Laptop Lift (Autodesk Fusion 360 design; units mm, degrees)
Autodesk Fusion 360 part; units mm, degrees
sketch "Sketch1" plane through (0, 0, 0) normal (0, 0, 1) x (1, 0, 0)
  line L0 (0, 0) -> (215, 0)
  line L1 (215, 0) -> (215, 180)
  line L2 (215, 180) -> (0, 180)
  line L3 (0, 180) -> (0, 0)
  line L4 (-17.5, 180) -> (232.5, 180)
  line L5 (232.5, 180) -> (232.5, 0)
  line L6 (232.5, 0) -> (-17.5, 0)
  line L7 (-17.5, 0) -> (-17.5, 180)
  line L8 (-17.5, 0) -> (0, 180)
  line L9 (232.5, 0) -> (215, 180)
  dimension "d1" = 215
  dimension "d2" = 180
  dimension "d3" = 250
  dimension "d4" = 180
  constraint horizontal L0
  constraint vertical L1
  constraint horizontal L2
  constraint vertical L3
  constraint coincident L0.start L3.end
  constraint horizontal L4
  constraint vertical L5
  constraint horizontal L6
  constraint vertical L7
  constraint collinear L2 L4
  constraint midpoint L0 L6
  measures "d1" distance of L1.end L2.end
  measures "d2" distance of L0.start L2.end
  measures "d3" distance of L4.start L4.end
  measures "d4" distance of L4.start L6.end
extrude "Extrude1" add sketch "Sketch1" along normal blind 3 contours L0 L1 L2 L3 L4 L6 | L3 L6 L8 | L1 L6 L9 makes body 1
fillet "Fillet1" radius 25 2 edges at (232.5, 0, 1.5) (-17.5, 0, 1.5) on bodies 1
sketch "Sketch5" plane through (0, 0, 3) normal (0, 0, 1) x (-1, 0, 0)
  arc A0 (14.8342, -27.4191) -> (-10.0484, 0) centre (-10.0484, -25) ccw
  line L0 (-10.0484, 0) -> (-204.9516, 0)
  arc A1 (-204.9516, 0) -> (-229.8342, -27.4191) centre (-204.9516, -25) ccw
  line L1 (-229.8342, -27.4191) -> (-215, -180)
  line L2 (-215, -180) -> (0, -180)
  line L3 (0, -180) -> (14.8342, -27.4191)
  arc A2 (17.8202, -27.7094) -> (-10.0484, 3) centre (-10.0484, -25) ccw
  line L4 (-10.0484, 3) -> (-204.9516, 3)
  arc A3 (-204.9516, 3) -> (-232.8202, -27.7094) centre (-204.9516, -25) ccw
  line L5 (-232.8202, -27.7094) -> (-217.7225, -183)
  line L6 (-217.7225, -183) -> (2.7225, -183)
  line L7 (2.7225, -183) -> (17.8202, -27.7094)
  line L8 (40, -180) -> (-310, -180)
  dimension "d21" = 3
  constraint horizontal L8
  constraint collinear L2 L8
extrude "Extrude4" add sketch "Sketch5" along normal blind 5 and the other way blind 3 contours A0 L0 A1 L1 L3 A2 L4 A3 L5 L7 L8 bodies 1
chamfer "Chamfer2" distance 80 distance2 4 2 edges at (216.5071, 180, 8) (-1.5071, 180, 8) measured on face at (75.0161, -1, 8) measured on face at (75.0161, -1, 8) on bodies 1
sketch "Sketch7" plane through (0, 0, 0) normal (0, 0, -1) x (1, 0, 0)
  line L0 (-3.0141, -180) -> (218.0141, -180)
  line L1 (218.0141, -180) -> (232.8202, -27.7094)
  arc A0 (232.8202, -27.7094) -> (204.9516, 3) centre (204.9516, -25) ccw
  line L2 (204.9516, 3) -> (10.0484, 3)
  arc A1 (10.0484, 3) -> (-17.8202, -27.7094) centre (10.0484, -25) ccw
  line L3 (-17.8202, -27.7094) -> (-3.0141, -180)
  line L4 (22, 3) -> (62, 3)
  line L5 (62, 3) -> (62, -147)
  line L6 (62, -147) -> (22, -147)
  line L7 (22, -147) -> (22, 3)
  line L8 (34.5, -122) -> (49.5, -122)
  line L9 (49.5, -122) -> (49.5, -107)
  line L10 (49.5, -107) -> (34.5, -107)
  line L11 (34.5, -107) -> (34.5, -122)
  line L12 (34.5, -82) -> (49.5, -82)
  line L13 (49.5, -82) -> (49.5, -67)
  line L14 (49.5, -67) -> (34.5, -67)
  line L15 (34.5, -67) -> (34.5, -82)
  line L16 (34.5, -42) -> (49.5, -42)
  line L17 (49.5, -42) -> (49.5, -27)
  line L18 (49.5, -27) -> (34.5, -27)
  line L19 (34.5, -27) -> (34.5, -42)
  line L20 (0, -312.52) -> (0, 100)
  line L21 (220, -311.5375) -> (220, 100.9826)
  line L22 (158, -147) -> (158, 3)
  line L23 (158, 3) -> (198, 3)
  line L24 (198, 3) -> (198, -147)
  line L25 (198, -147) -> (158, -147)
  line L26 (170.5, -27) -> (170.5, -42)
  line L27 (170.5, -42) -> (185.5, -42)
  line L28 (185.5, -27) -> (170.5, -27)
  line L29 (185.5, -42) -> (185.5, -27)
  line L30 (170.5, -67) -> (170.5, -82)
  line L31 (170.5, -82) -> (185.5, -82)
  line L32 (185.5, -67) -> (170.5, -67)
  line L33 (185.5, -82) -> (185.5, -67)
  line L34 (170.5, -107) -> (170.5, -122)
  line L35 (170.5, -122) -> (185.5, -122)
  line L36 (185.5, -107) -> (170.5, -107)
  line L37 (185.5, -122) -> (185.5, -107)
  line L38 (198, -147) -> (22, -147)
  line L39 (22, -147) -> (22, -122)
  line L40 (22, -122) -> (198, -122)
  line L41 (198, -122) -> (198, -147)
  line L42 (198, 3) -> (22, 3)
  line L43 (22, 3) -> (22, -22)
  line L44 (22, -22) -> (198, -22)
  line L45 (198, -22) -> (198, 3)
  point P0 (215, -180)
  point P1 (0, -180)
  dimension "d28" = 40
  dimension "d29" = 150
  dimension "d30" = 15
  dimension "d31" = 15
  dimension "d32" = 12.5
  dimension "d33" = 15
  dimension "d34" = 15
  dimension "d35" = 15
  dimension "d36" = 15
  dimension "d37" = 25
  dimension "d38" = 25
  dimension "d39" = 25
  dimension "d40" = 22
  dimension "d41" = 12.5
  dimension "d42" = 12.5
  dimension "d43" = 40
  dimension "d44" = 150
  dimension "d45" = 15
  dimension "d46" = 15
  dimension "d47" = 12.5
  dimension "d48" = 15
  dimension "d49" = 15
  dimension "d50" = 15
  dimension "d51" = 15
  dimension "d52" = 25
  dimension "d53" = 25
  dimension "d54" = 25
  dimension "d55" = 12.5
  dimension "d56" = 12.5
  dimension "d57" = 22
  dimension "d60" = 25
  dimension "d61" = 25
  constraint horizontal L4
  constraint vertical L5
  constraint horizontal L6
  constraint vertical L7
  constraint coincident L2 L4.start
  constraint horizontal L8
  constraint vertical L9
  constraint horizontal L10
  constraint vertical L11
  constraint horizontal L12
  constraint vertical L13
  constraint horizontal L14
  constraint vertical L15
  constraint horizontal L16
  constraint vertical L17
  constraint horizontal L18
  constraint vertical L19
  constraint vertical L20
  constraint vertical L21
  constraint horizontal L23
  constraint vertical L24
  constraint horizontal L25
  constraint vertical L22
  constraint horizontal L35
  constraint vertical L37
  constraint horizontal L36
  constraint vertical L34
  constraint horizontal L31
  constraint vertical L33
  constraint horizontal L32
  constraint vertical L30
  constraint horizontal L27
  constraint vertical L29
  constraint horizontal L28
  constraint vertical L26
  constraint horizontal L38
  constraint vertical L39
  constraint horizontal L40
  constraint vertical L41
  constraint coincident L7 L39.end
  constraint horizontal L42
  constraint vertical L43
  constraint horizontal L44
  constraint vertical L45
  constraint coincident L7 L43.end
  measures "d28" distance of L4.start L4.end
  measures "d29" distance of L4.start L6.end
  measures "d30" distance of L8.start L8.end
  measures "d31" distance of L8.start L10.end
  measures "d32" distance of L7 L11
  measures "d33" distance of L12.end L12.start
  measures "d34" distance of L12.start L14.end
  measures "d35" distance of L16.end L16.start
  measures "d36" distance of L18.end L16.start
  measures "d37" distance of L14 L16
  measures "d38" distance of L10 L12
  measures "d39" distance of L6 L8
  measures "d40" distance of L7 L20
  measures "d41" distance of L7 L15
  measures "d42" distance of L7 L19
  measures "d43" distance of L22.end L23.end
  measures "d44" distance of L22.end L22.start
  measures "d45" distance of L35.end L34.end
  measures "d46" distance of L34.end L34.start
  measures "d47" distance of L22 L34
  measures "d48" distance of L31.end L30.end
  measures "d49" distance of L30.start L30.end
  measures "d50" distance of L26.end L27.end
  measures "d51" distance of L26.end L26.start
  measures "d52" distance of L27 L32
  measures "d53" distance of L31 L36
  measures "d54" distance of L25 L35
  measures "d55" distance of L22 L30
  measures "d56" distance of L22 L26
  measures "d57" distance of L21 L24
  measures "d60" distance of L24.end L40.end
  measures "d61" distance of L23.end L44.end
extrude "Extrude6" add sketch "Sketch7" along normal blind 5 separate body contours L2 L4 L5 L7 L42 L43 L44 | L2 L5 L22 L42 L44 | L5 L7 L9 L10 L11 L40 L44 | L2 L22 L23 L24 L42 L44 L45 | L5 L6 L7 L8 L38 L39 L40 | L22 L24 L34 L36 L37 L40 L44 | L5 L22 L38 L40 | L8 L9 L10 L11 L40 | L22 L24 L25 L35 L38 L40 L41 | L34 L35 L36 L37 L40 | L12 L13 L14 L15 | L16 L17 L18 L19 | L26 L27 L28 L29 | L30 L31 L32 L33 makes body 2
sketch "Sketch8" plane through (22, 0, 0) normal (-1, 0, 0) x (0, -1, 0)
  line L0 (3, 0) -> (-147, 0)
  line L1 (-147, 0) -> (-147, -5)
  line L2 (-147, -5) -> (3, -5)
  line L3 (3, -5) -> (3, 0)
  line L4 (3, -5) -> (-132.9462, -68.3927)
  line L5 (3, -5) -> (153, -5) construction
  line L6 (-132.9462, -68.3927) -> (-135.0593, -63.8612)
  line L7 (-132.9462, -68.3927) -> (-127.9462, -68.3927) construction
  line L8 (-135.0593, -63.8612) -> (-8.831, -5)
  dimension "d65" = 150
  dimension "d67" = 25
  dimension "d69" = 5
  dimension "d70" = 90
  constraint horizontal L5
  constraint coincident L2.end L3.start
  constraint horizontal L7
  constraint coincident L2 L8.end
  constraint perpendicular L6 L8
  measures "d65" distance of L2.end L4.end
  measures "d67" angle of L2 L4
  measures "d69" distance of L4.end L6.end
  measures "d70" angle of L4 L6
ref_plane "WorkPlane1" through (-18, 0, 0) normal (1, 0, 0) x (0, 1, 0)
sketch "Sketch12" plane through (-18, 0, 0) normal (1, 0, 0) x (0, 1, 0)
  line L0 (-3, 0) -> (132.9462, -63.3927)
  line L1 (-3, 0) -> (147, 0) construction
  line L2 (132.9462, -63.3927) -> (135.0593, -58.8612)
  line L3 (135.0593, -58.8612) -> (5, 0)
  line L4 (5, 0) -> (-3, 0)
  line L5 (135.0593, -58.8612) -> (135.0593, 0)
  line L6 (135.0593, 0) -> (130.0593, 0)
  line L7 (130.0593, -56.5983) -> (130.0593, 0)
  dimension "d72" = 25
  dimension "d73" = 150
  dimension "d74" = 5
  dimension "d78" = 5
  constraint horizontal L1
  constraint perpendicular L0 L2
  constraint coincident L1 L3.end
  constraint coincident L1 L5.end
  constraint perpendicular L1 L5
  constraint perpendicular L5 L6
  constraint coincident L3 L7.start
  constraint perpendicular L1 L7
  measures "d72" angle of L0 L1
  measures "d73" distance of L0.start L0.end
  measures "d74" distance of L0.end L2.end
  measures "d78" distance of L5.end L6.end
extrude "Extrude7" add sketch "Sketch12" along normal blind 40 from surface at 40 separate body makes body 3
sketch "Sketch13" plane through (0, 0, 0) normal (0, 0, 1) x (-1, 0, 0)
  line L0 (-22, -5) -> (-22, 3)
  line L1 (-22, 3) -> (-62, 3)
  line L2 (-62, 3) -> (-62, -5)
  line L3 (-62, -5) -> (-22, -5)
  line L4 (-22, -5) -> (-32, -5)
  line L5 (-32, -5) -> (-32, 0)
  line L6 (-32, 0) -> (-22, 0)
  line L7 (-22, 0) -> (-22, -5)
  line L8 (-62, -5) -> (-52, -5)
  line L9 (-52, -5) -> (-52, 0)
  line L10 (-52, 0) -> (-62, 0)
  line L11 (-62, 0) -> (-62, -5)
  dimension "d79" = 10
  dimension "d80" = 5
  dimension "d81" = 10
  dimension "d82" = 5
  constraint horizontal L4
  constraint vertical L5
  constraint horizontal L6
  constraint vertical L7
  constraint coincident L0.start L3.end
  constraint horizontal L8
  constraint vertical L9
  constraint horizontal L10
  constraint vertical L11
  constraint coincident L2.end L3.start
  measures "d79" distance of L0.start L4.end
  measures "d80" distance of L0.start L6.end
  measures "d81" distance of L2.end L8.end
  measures "d82" distance of L2.end L10.end
extrude "Extrude8" cut sketch "Sketch13" along normal blind 10 contours L0 L3 L4 L5 L6 L7 | L2 L3 L8 L9 L10 L11 bodies 1
extrude "Extrude9" add sketch "Sketch13" along normal blind 3 contours L0 L3 L4 L5 L6 L7 | L2 L3 L8 L9 L10 L11 bodies 3
sketch "Sketch14" plane through (0, 0, 0) normal (0, 0, 1) x (-1, 0, 0)
  line L0 (-22, -135.0593) -> (-22, -130.0593)
  line L1 (-22, -130.0593) -> (-62, -130.0593)
  line L2 (-62, -130.0593) -> (-62, -135.0593)
  line L3 (-62, -135.0593) -> (-22, -135.0593)
  line L4 (-22, -135.0593) -> (-32, -135.0593)
  line L5 (-32, -135.0593) -> (-32, -130.0593)
  line L6 (-32, -130.0593) -> (-22, -130.0593)
  line L7 (-22, -130.0593) -> (-22, -135.0593)
  line L8 (-62, -135.0593) -> (-52, -135.0593)
  line L9 (-52, -135.0593) -> (-52, -130.0593)
  line L10 (-52, -130.0593) -> (-62, -130.0593)
  line L11 (-62, -130.0593) -> (-62, -135.0593)
  line L12 (-32, -130.0593) -> (-22, -130.0593)
  line L13 (-62, -135.0593) -> (-52, -135.0593)
  line L14 (-52, -130.0593) -> (-62, -130.0593)
  line L15 (-52, -135.0593) -> (-52, -130.0593)
  line L16 (-22, -135.0593) -> (-22, -130.0593)
  line L17 (-22, -135.0593) -> (-32, -135.0593)
  line L18 (-62, -130.0593) -> (-62, -135.0593)
  line L19 (-62, -135.0593) -> (-22, -135.0593)
  line L20 (-32, -135.0593) -> (-32, -130.0593)
  line L21 (-62, -130.0593) -> (-62, -135.0593)
  line L22 (-22, -130.0593) -> (-22, -135.0593)
  line L23 (-22, -130.0593) -> (-62, -130.0593)
  dimension "d87" = 10
  dimension "d88" = 5
  dimension "d89" = 10
  dimension "d90" = 5
  dimension "d95" = 10
  dimension "d96" = 5
  dimension "d97" = 10
  dimension "d98" = 5
  constraint horizontal L4
  constraint vertical L5
  constraint horizontal L6
  constraint vertical L7
  constraint coincident L0.start L3.end
  constraint horizontal L8
  constraint vertical L9
  constraint horizontal L10
  constraint vertical L11
  constraint coincident L2.end L3.start
  constraint horizontal L17
  constraint vertical L20
  constraint horizontal L12
  constraint vertical L22
  constraint horizontal L13
  constraint vertical L15
  constraint horizontal L14
  constraint vertical L21
  measures "d87" distance of L0.start L4.end
  measures "d88" distance of L0.start L0.end
  measures "d89" distance of L2.end L8.end
  measures "d90" distance of L2.end L1.end
  measures "d95" distance of L0.start L4.end
  measures "d96" distance of L0.start L0.end
  measures "d97" distance of L2.end L8.end
  measures "d98" distance of L2.end L1.end
extrude "Extrude10" cut sketch "Sketch14" along normal blind 30 contours L0 L1 L3 L4 L5 L6 L7 L12 L16 L17 L19 L20 L22 L23 | L1 L2 L3 L8 L9 L10 L11 L13 L14 L15 L18 L19 L21 L23 bodies 1
extrude "Extrude11" add sketch "Sketch14" along normal blind 3 contours L0 L1 L3 L4 L5 L6 L7 L12 L16 L17 L19 L20 L22 L23 | L1 L2 L3 L8 L9 L10 L11 L13 L14 L15 L18 L19 L21 L23 bodies 3
ref_plane "WorkPlane2" through (233, 0, 0) normal (1, 0, 0) x (0, 1, 0)
hidden bodies 2 3
